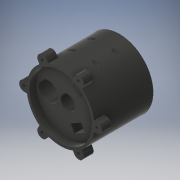
# Autodesk Inventor part: TA02
Saved by Autodesk Inventor 2017 (Build 210142000, 142)
## iProperties
Created: 2018-10-09
Part Number: TA02
Material: ABS Plastic
Document SubType Name: Modeling
Designer: Zach
Density: 1.06 g/cm^3
Appearance: Smooth - Black
Author: Zach
Autodesk Inventor part; units mm, degrees
ref_plane "YZ Plane" through (0, 0, 0) normal (1, 0, 0) x (0, 1, 0)
ref_plane "XZ Plane" through (0, 0, 0) normal (0, 1, 0) x (-1, 0, 0)
ref_plane "XY Plane" through (0, 0, 0) normal (0, 0, 1) x (1, 0, 0)
sketch "Sketch1" plane through (0, 0, 0) normal (0, 0, 1) x (1, 0, 0)
  circle A0 centre (0, 0) radius 68.75
  circle A1 centre (0, 0) radius 15
  circle A2 centre (-40, 0) radius 4
  line L0 (-49, 9) -> (-31, 9) construction
  line L1 (-31, 9) -> (-31, -9) construction
  line L2 (-31, -9) -> (-49, -9) construction
  line L3 (-49, -9) -> (-49, 9) construction
  circle A3 centre (-49, 9) radius 2
  circle A4 centre (-31, 9) radius 2
  circle A5 centre (-31, -9) radius 2
  circle A6 centre (-49, -9) radius 2
  circle A7 centre (20, 34.641) radius 3.5
  line L4 (0, 0) -> (-40, 0) construction
  line L5 (0, 0) -> (20, 34.641) construction
  line L6 (0, 0) -> (20, -34.641) construction
  circle A8 centre (20, -34.641) radius 3.5
  point P0 (-49, 0)
  point P1 (-40, 9)
  dimension "d0" = 137.5
  dimension "d1" = 30
  dimension "d2" = 8
  dimension "d3" = 40
  dimension "d4" = 18
  dimension "d5" = 18
  dimension "d6" = 4
  dimension "d7" = 4
  dimension "d8" = 4
  dimension "d9" = 4
  dimension "d10" = 7
  dimension "d11" = 40
  dimension "d12" = 120
  dimension "d13" = 40
  dimension "d14" = 7
  dimension "d15" = 120
  constraints: 14 end point, 9 centre point, 8 coincident, 2 horizontal, 2 horizontal alignment, 2 midpoint, 2 parallel, 1 perpendicular, 1 vertical alignment
  measures "d0" diameter of A0
  measures "d1" diameter of A1
  measures "d2" diameter of A2
  measures "d3" distance of L4.end point (0, 0)
  measures "d4" distance of L1.end L2.end
  measures "d5" distance of L0.end L1.end
  measures "d6" diameter of A3
  measures "d7" diameter of A4
  measures "d8" diameter of A5
  measures "d9" diameter of A6
  measures "d10" diameter of A7
  measures "d11" distance of L5.start L5.end
  measures "d12" angle of L5 L4
  measures "d13" distance of L5.start L6.end
  measures "d14" diameter of A8
  measures "d15" angle of L4 L6
extrude "Extrusion1" add sketch "Sketch1" along normal blind 5
sketch "Sketch2" plane through (0, 0, 5) normal (0, 0, 1) x (1, 0, 0)
  circle A0 centre (0, 0) radius 68.75 projected
  circle A1 centre (0, 0) radius 63.75
  dimension "d18" = 5
  constraints: 1 centre point, 1 coincident
  measures "d18" radial gap between concentric circles of A0 A1
extrude "Extrusion2" add sketch "Sketch2" along normal blind 115
sketch "Sketch3" plane through (0, 0, 5) normal (0, 0, 1) x (1, 0, 0)
  circle A0 centre (-40, 0) radius 4 projected
  circle A1 centre (0, 0) radius 15 projected
  circle A2 centre (20, 34.641) radius 3.5 projected
  circle A3 centre (20, -34.641) radius 3.5 projected
  circle A4 centre (-40, 0) radius 20
  line L0 (26.8253, 21.4628) -> (5.1747, 33.9628)
  line L1 (5.1747, 33.9628) -> (13.1747, 47.8192)
  line L2 (13.1747, 47.8192) -> (34.8253, 35.3192)
  line L3 (34.8253, 35.3192) -> (26.8253, 21.4628)
  line L4 (26.8253, 21.4628) -> (13.1747, 47.8192) construction
  line L5 (5.1747, 33.9628) -> (34.8253, 35.3192) construction
  line L6 (0, 0) -> (-40, 0) construction
  line L7 (5.1747, -33.9628) -> (26.8253, -21.4628)
  line L8 (26.8253, -21.4628) -> (34.8253, -35.3192)
  line L9 (34.8253, -35.3192) -> (13.1747, -47.8192)
  line L10 (13.1747, -47.8192) -> (5.1747, -33.9628)
  circle A5 centre (0, 0) radius 63.75 projected
  dimension "d21" = 40
  dimension "d23" = 120
  dimension "d24" = 16
  dimension "d25" = 25
  dimension "d28" = 120
  constraints: 22 end point, 2 midpoint, 2 parallel, 1 centre point, 1 coincident, 1 horizontal, 1 perpendicular, 9 other
  measures "d21" diameter of A4
  measures "d23" angle of L6 L1
  measures "d24" distance of L0.end L1.end
  measures "d25" distance of L1.end L2.end
extrude "Extrusion3" add sketch "Sketch3" along normal blind 100 contours A5
sketch "Sketch4" plane through (0, 0, 105) normal (0, 0, 1) x (1, 0, 0)
  circle A0 centre (50, 0) radius 3
  circle A1 centre (-25, 43.3013) radius 3
  circle A2 centre (-25, -43.3013) radius 3
  circle A3 centre (50, 0) radius 15
  circle A4 centre (-25, 43.3013) radius 15
  circle A5 centre (-25, -43.3013) radius 15
  point P0 (0, 0)
  dimension "d32" = 6
  dimension "d33" = 50
  dimension "d36" = 360
  dimension "d38" = 30
  dimension "d39" = 30
  dimension "d40" = 30
  constraints: 6 centre point, 3 coincident, 1 horizontal alignment, 7 other
  measures "d32" diameter of A0
  measures "d33" distance of A0.centre point (0, 0)
  measures "d38" diameter of A3
  measures "d39" diameter of A4
  measures "d40" diameter of A5
extrude "Extrusion4" add sketch "Sketch4" along normal blind 15
sketch "Sketch6" plane through (-40, 0, 5) normal (0, 0, 1) x (1, 0, 0)
  circle A0 centre (0, 0) radius 4 projected
  circle A1 centre (0, 0) radius 16.5
  circle A2 centre (0, 0) radius 20 projected
  point P0 (40, 0)
  point P1 (20, 0)
  dimension "d46" = 33
  constraints: 1 centre point, 1 coincident, 1 horizontal alignment
  measures "d46" diameter of A1
extrude "Extrusion6" add sketch "Sketch6" along normal blind 40 contours A2
sketch "Sketch7" plane through (0, 0, 120) normal (0, 0, 1) x (1, 0, 0)
  circle A0 centre (37, 64.0859) radius 10
  line L0 (28.3397, 69.0859) -> (25.3492, 63.906)
  line L1 (45.6603, 59.0859) -> (42.6697, 53.906)
  circle A1 centre (0, 0) radius 68.75 construction
  line L2 (0, 0) -> (37, 64.0859) construction
  line L3 (25.3492, 63.906) -> (42.6697, 53.906)
  circle A2 centre (20, 34.641) radius 3.5 projected
  circle A3 centre (37, 64.0859) radius 3
  circle A4 centre (-37, 64.0859) radius 10
  line L4 (-45.6603, 59.0859) -> (-42.6697, 53.906)
  line L5 (-28.3397, 69.0859) -> (-25.3492, 63.906)
  line L6 (-42.6697, 53.906) -> (-25.3492, 63.906)
  circle A5 centre (-37, 64.0859) radius 3
  circle A6 centre (-74, 0) radius 10
  line L7 (-74, -10) -> (-68.0188, -10)
  line L8 (-74, 10) -> (-68.0188, 10)
  line L9 (-68.0188, -10) -> (-68.0188, 10)
  circle A7 centre (-74, 0) radius 3
  circle A8 centre (-37, -64.0859) radius 10
  line L10 (-28.3397, -69.0859) -> (-25.3492, -63.906)
  line L11 (-45.6603, -59.0859) -> (-42.6697, -53.906)
  line L12 (-25.3492, -63.906) -> (-42.6697, -53.906)
  circle A9 centre (-37, -64.0859) radius 3
  circle A10 centre (37, -64.0859) radius 10
  line L13 (45.6603, -59.0859) -> (42.6697, -53.906)
  line L14 (28.3397, -69.0859) -> (25.3492, -63.906)
  line L15 (42.6697, -53.906) -> (25.3492, -63.906)
  circle A11 centre (37, -64.0859) radius 3
  circle A12 centre (74, 0) radius 10
  line L16 (74, 10) -> (68.0188, 10)
  line L17 (74, -10) -> (68.0188, -10)
  line L18 (68.0188, 10) -> (68.0188, -10)
  circle A13 centre (74, 0) radius 3
  dimension "d49" = 20
  dimension "d52" = 74
  dimension "d53" = 6
  dimension "d56" = 360
  constraints: 38 end point, 14 point on circle, 12 centre point, 6 coincident, 2 parallel, 2 tangent, 1 point on line, 67 other
  measures "d49" diameter of A0
  measures "d52" distance of L2.start L2.end
  measures "d53" diameter of A3
extrude "Extrusion7" add sketch "Sketch7" against normal blind 20 contours A0 L3 | A0 L3 L0 | L1 L3 A0 | L3 A0 | A4 L6 | A4 L5 L6 | A4 L6 | A4 L6 L4 | A6 L9 | L8 L9 A6 | A6 L9 L7 | A6 L9 | A8 L12 | L11 L12 A8 | A8 L12 L10 | A8 L12 | A10 L15 | A10 L15 L13 | L14 L15 A10 | L15 A10 | A12 L18 | A12 L18 L16 | L17 L18 A12 | L18 A12
sketch "Sketch8" plane through (0, 0, 105) normal (0, 0, 1) x (1, 0, 0)
  circle A0 centre (0, 0) radius 63.75
  dimension "d62" = 127.5
  constraints: 1 centre point, 1 coincident
  measures "d62" diameter of A0
extrude "Extrusion8" cut sketch "Sketch8" along normal through all
sketch "Sketch13" plane through (0, 0, 0) normal (1, 0, 0) x (0, 1, 0)
  circle A0 centre (-63.75, 72.5) radius 3
  circle A1 centre (-63.75, 32.5) radius 3
  circle A2 centre (63.75, 72.5) radius 3
  circle A3 centre (63.75, 32.5) radius 3
  line L0 (-63.75, 32.5) -> (-63.75, 72.5) construction
  line L1 (63.75, 32.5) -> (63.75, 72.5) construction
  line L2 (-68.75, 0) -> (-68.75, 120) projected
  line L3 (68.75, 0) -> (68.75, 120) projected
  line L4 (0, 0) -> (0, 105)
  line L5 (-15, 105) -> (15, 105) projected
  point P0 (-63.75, 52.5)
  point P1 (63.75, 52.5)
  point P2 (0, 52.5)
  dimension "d69" = 6
  dimension "d70" = 6
  dimension "d71" = 6
  dimension "d72" = 6
  dimension "d73" = 40
  dimension "d74" = 5
  dimension "d75" = 5
  constraints: 6 end point, 4 centre point, 4 midpoint, 3 horizontal alignment, 3 vertical, 2 vertical alignment
  measures "d69" diameter of A0
  measures "d70" diameter of A1
  measures "d71" diameter of A2
  measures "d72" diameter of A3
  measures "d73" distance of L0.start L0.end
  measures "d74" distance between parallel lines of L2 L0
  measures "d75" distance between parallel lines of L3 L1
extrude "Extrusion11" cut sketch "Sketch13" along normal through all both and the other way through all
body "Solid1"
